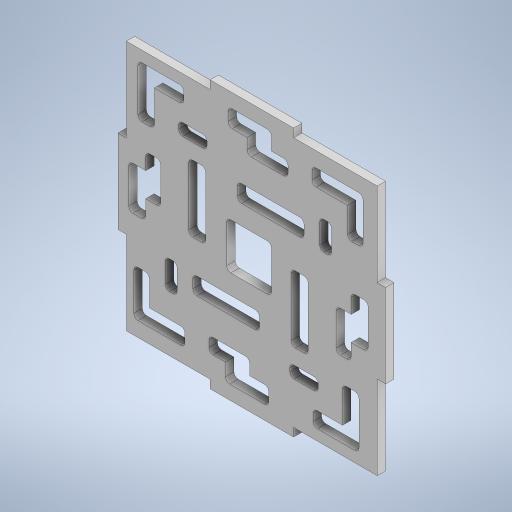
# Autodesk Inventor part: Pièce Ve2
Saved by Autodesk Inventor 2023 (Build 270158000, 158)
## iProperties
Created: 2025-01-14
Part Number: Pièce Ve2
Material: Générique
Document SubType Name: Modeling
Designer: kfadieieva
Density: 1 g/cm^3
Appearance: Par défaut
Author: kfadieieva
Autodesk Inventor part; units mm, degrees
ref_plane "YZ Plane" through (0, 0, 0) normal (1, 0, 0) x (0, 1, 0)
ref_plane "XZ Plane" through (0, 0, 0) normal (0, 1, 0) x (-1, 0, 0)
ref_plane "XY Plane" through (0, 0, 0) normal (0, 0, 1) x (1, 0, 0)
sketch "Esquisse1" plane through (0, 0, 0) normal (0, 0, 1) x (1, 0, 0)
  line L0 (0, 60) -> (-3, 60)
  line L1 (-3, 60) -> (-3, 30)
  line L2 (-3, 30) -> (0, 30)
  line L3 (90, 60) -> (93, 60)
  line L4 (93, 60) -> (93, 30)
  line L5 (93, 30) -> (90, 30)
  line L6 (60, 90) -> (60, 93)
  line L7 (60, 93) -> (30, 93)
  line L8 (30, 93) -> (30, 90)
  line L9 (30, 0) -> (30, -3)
  line L10 (30, -3) -> (60, -3)
  line L11 (60, -3) -> (60, 0)
  line L12 (0, 0) -> (30, 0)
  line L13 (60, 0) -> (90, 0)
  line L14 (90, 90) -> (60, 90)
  line L15 (30, 90) -> (0, 90)
  line L16 (90, 0) -> (90, 30)
  line L17 (90, 60) -> (90, 90)
  line L18 (0, 90) -> (0, 60)
  line L19 (0, 30) -> (0, 0)
  dimension "d0" = 90
  dimension "d1" = 90
  dimension "d6" = 3
  constraints: 40 end point, 13 perpendicular, 8 parallel, 3 equal length, 3 horizontal, 2 point on line, 2 vertical
  measures "d0" distance of L15.end L12.start
  measures "d1" distance of L12.start L13.end
  measures "d6" distance of L0.start L0.end
extrude "Extrusion1" add sketch "Esquisse1" along normal blind 3
sketch "Esquisse2" plane through (0, 0, 3) normal (0, 0, 1) x (1, 0, 0)
  line L0 (5.6535, 86.1061) -> (19.1192, 86.1061)
  line L1 (20.6192, 84.6061) -> (20.6192, 82.0558)
  line L2 (19.1192, 80.5558) -> (10.0738, 80.5558)
  line L3 (4.1535, 80.5558) -> (4.1535, 84.6061)
  line L4 (10.0738, 80.5558) -> (10.0738, 69.2903)
  line L5 (8.5738, 67.7903) -> (5.6535, 67.7903)
  line L6 (4.1535, 69.2903) -> (4.1535, 81.8509)
  line L7 (20.2692, 74.8206) -> (27.4446, 74.8206)
  line L8 (28.9446, 73.3206) -> (28.9446, 72.0654)
  line L9 (27.4446, 70.5654) -> (20.2692, 70.5654)
  line L10 (18.7692, 72.0654) -> (18.7692, 73.3206)
  line L11 (38.0299, 87.9562) -> (50.5706, 87.9562)
  line L12 (52.0706, 86.4562) -> (52.0706, 81.8509)
  line L13 (43.3752, 81.8509) -> (38.0299, 81.8509)
  line L14 (36.5299, 83.3509) -> (36.5299, 86.4562)
  line L15 (52.0706, 81.8509) -> (56.4909, 81.8509)
  line L16 (57.9909, 80.3509) -> (57.9909, 77.9857)
  line L17 (56.4909, 76.4857) -> (44.8752, 76.4857)
  line L18 (43.3752, 77.9857) -> (43.3752, 81.8509)
  arc A0 (5.6535, 86.1061) -> (4.1535, 84.6061) centre (5.6535, 84.6061) ccw
  arc A1 (19.1192, 80.5558) -> (20.6192, 82.0558) centre (19.1192, 82.0558) ccw
  arc A2 (20.6192, 84.6061) -> (19.1192, 86.1061) centre (19.1192, 84.6061) ccw
  arc A3 (20.2692, 74.8206) -> (18.7692, 73.3206) centre (20.2692, 73.3206) ccw
  arc A4 (18.7692, 72.0654) -> (20.2692, 70.5654) centre (20.2692, 72.0654) ccw
  arc A5 (28.9446, 73.3206) -> (27.4446, 74.8206) centre (27.4446, 73.3206) ccw
  arc A6 (27.4446, 70.5654) -> (28.9446, 72.0654) centre (27.4446, 72.0654) ccw
  arc A7 (8.5738, 67.7903) -> (10.0738, 69.2903) centre (8.5738, 69.2903) ccw
  arc A8 (4.1535, 69.2903) -> (5.6535, 67.7903) centre (5.6535, 69.2903) ccw
  arc A9 (43.3752, 77.9857) -> (44.8752, 76.4857) centre (44.8752, 77.9857) ccw
  arc A10 (38.0299, 87.9562) -> (36.5299, 86.4562) centre (38.0299, 86.4562) ccw
  arc A11 (36.5299, 83.3509) -> (38.0299, 81.8509) centre (38.0299, 83.3509) ccw
  arc A12 (56.4909, 76.4857) -> (57.9909, 77.9857) centre (56.4909, 77.9857) ccw
  arc A13 (57.9909, 80.3509) -> (56.4909, 81.8509) centre (56.4909, 80.3509) ccw
  arc A14 (52.0706, 86.4562) -> (50.5706, 87.9562) centre (50.5706, 86.4562) ccw
  line L19 (60, 93) -> (30, 93) projected
  line L20 (93, 30) -> (93, 60) projected
  line L21 (-3, 60) -> (-3, 30) projected
  line L22 (30, -3) -> (60, -3) projected
  line L23 (83.4207, 68.1953) -> (80.8704, 68.1953)
  arc A15 (83.4207, 68.1953) -> (84.9207, 69.6953) centre (83.4207, 69.6953) ccw
  arc A16 (79.3704, 69.6953) -> (80.8704, 68.1953) centre (80.8704, 69.6953) ccw
  line L24 (70.88, 70.0454) -> (72.1352, 70.0454)
  arc A17 (73.6352, 68.5454) -> (72.1352, 70.0454) centre (72.1352, 68.5454) ccw
  arc A18 (70.88, 70.0454) -> (69.38, 68.5454) centre (70.88, 68.5454) ccw
  line L25 (73.6352, 68.5454) -> (73.6352, 61.37)
  line L26 (69.38, 61.37) -> (69.38, 68.5454)
  arc A19 (72.1352, 59.87) -> (73.6352, 61.37) centre (72.1352, 61.37) ccw
  line L27 (72.1352, 59.87) -> (70.88, 59.87)
  arc A20 (69.38, 61.37) -> (70.88, 59.87) centre (70.88, 61.37) ccw
  line L28 (66.6049, 80.2408) -> (66.6049, 83.1611)
  arc A21 (66.6049, 80.2408) -> (68.1049, 78.7408) centre (68.1049, 80.2408) ccw
  arc A22 (68.1049, 84.6611) -> (66.6049, 83.1611) centre (68.1049, 83.1611) ccw
  line L29 (80.6655, 45.4393) -> (80.6655, 50.7846)
  line L30 (80.6655, 36.744) -> (80.6655, 32.3237)
  line L31 (79.1655, 30.8237) -> (76.8002, 30.8237)
  line L32 (75.3002, 32.3237) -> (75.3002, 43.9393)
  line L33 (76.8002, 45.4393) -> (80.6655, 45.4393)
  arc A23 (79.1655, 30.8237) -> (80.6655, 32.3237) centre (79.1655, 32.3237) ccw
  arc A24 (76.8002, 45.4393) -> (75.3002, 43.9393) centre (76.8002, 43.9393) ccw
  arc A25 (75.3002, 32.3237) -> (76.8002, 30.8237) centre (76.8002, 32.3237) ccw
  line L34 (84.9207, 83.1611) -> (84.9207, 69.6953)
  line L35 (79.3704, 69.6953) -> (79.3704, 78.7408)
  line L36 (79.3704, 84.6611) -> (83.4207, 84.6611)
  line L37 (79.3704, 78.7408) -> (68.1049, 78.7408)
  line L38 (68.1049, 84.6611) -> (80.6655, 84.6611)
  arc A26 (84.9207, 83.1611) -> (83.4207, 84.6611) centre (83.4207, 83.1611) ccw
  line L39 (86.7707, 50.7846) -> (86.7707, 38.244)
  line L40 (85.2707, 36.744) -> (80.6655, 36.744)
  line L41 (82.1655, 52.2846) -> (85.2707, 52.2846)
  arc A27 (82.1655, 52.2846) -> (80.6655, 50.7846) centre (82.1655, 50.7846) ccw
  arc A28 (86.7707, 50.7846) -> (85.2707, 52.2846) centre (85.2707, 50.7846) ccw
  arc A29 (85.2707, 36.744) -> (86.7707, 38.244) centre (85.2707, 38.244) ccw
  line L42 (67.0099, 5.3939) -> (67.0099, 7.9442)
  arc A30 (67.0099, 5.3939) -> (68.5099, 3.8939) centre (68.5099, 5.3939) ccw
  arc A31 (68.5099, 9.4442) -> (67.0099, 7.9442) centre (68.5099, 7.9442) ccw
  line L43 (68.86, 17.9346) -> (68.86, 16.6794)
  arc A32 (67.36, 15.1794) -> (68.86, 16.6794) centre (67.36, 16.6794) ccw
  arc A33 (68.86, 17.9346) -> (67.36, 19.4346) centre (67.36, 17.9346) ccw
  line L44 (67.36, 15.1794) -> (60.1846, 15.1794)
  line L45 (60.1846, 19.4346) -> (67.36, 19.4346)
  arc A34 (58.6846, 16.6794) -> (60.1846, 15.1794) centre (60.1846, 16.6794) ccw
  line L46 (58.6846, 16.6794) -> (58.6846, 17.9346)
  arc A35 (60.1846, 19.4346) -> (58.6846, 17.9346) centre (60.1846, 17.9346) ccw
  line L47 (79.0554, 22.2097) -> (81.9756, 22.2097)
  arc A36 (79.0554, 22.2097) -> (77.5554, 20.7097) centre (79.0554, 20.7097) ccw
  arc A37 (83.4756, 20.7097) -> (81.9756, 22.2097) centre (81.9756, 20.7097) ccw
  line L48 (44.2539, 8.1491) -> (49.5992, 8.1491)
  line L49 (35.5585, 8.1491) -> (31.1383, 8.1491)
  line L50 (29.6383, 9.6491) -> (29.6383, 12.0143)
  line L51 (31.1383, 13.5143) -> (42.7539, 13.5143)
  line L52 (44.2539, 12.0143) -> (44.2539, 8.1491)
  arc A38 (29.6383, 9.6491) -> (31.1383, 8.1491) centre (31.1383, 9.6491) ccw
  arc A39 (44.2539, 12.0143) -> (42.7539, 13.5143) centre (42.7539, 12.0143) ccw
  arc A40 (31.1383, 13.5143) -> (29.6383, 12.0143) centre (31.1383, 12.0143) ccw
  line L53 (81.9756, 3.8939) -> (68.5099, 3.8939)
  line L54 (68.5099, 9.4442) -> (77.5554, 9.4442)
  line L55 (83.4756, 9.4442) -> (83.4756, 5.3939)
  line L56 (77.5554, 9.4442) -> (77.5554, 20.7097)
  line L57 (83.4756, 20.7097) -> (83.4756, 8.1491)
  arc A41 (81.9756, 3.8939) -> (83.4756, 5.3939) centre (81.9756, 5.3939) ccw
  line L58 (49.5992, 2.0438) -> (37.0585, 2.0438)
  line L59 (35.5585, 3.5438) -> (35.5585, 8.1491)
  line L60 (51.0992, 6.6491) -> (51.0992, 3.5438)
  arc A42 (51.0992, 6.6491) -> (49.5992, 8.1491) centre (49.5992, 6.6491) ccw
  arc A43 (49.5992, 2.0438) -> (51.0992, 3.5438) centre (49.5992, 3.5438) ccw
  arc A44 (35.5585, 3.5438) -> (37.0585, 2.0438) centre (37.0585, 3.5438) ccw
  line L61 (4.2085, 21.8047) -> (6.7587, 21.8047)
  arc A45 (4.2085, 21.8047) -> (2.7085, 20.3047) centre (4.2085, 20.3047) ccw
  arc A46 (8.2587, 20.3047) -> (6.7587, 21.8047) centre (6.7587, 20.3047) ccw
  line L62 (16.7492, 19.9546) -> (15.494, 19.9546)
  arc A47 (13.994, 21.4546) -> (15.494, 19.9546) centre (15.494, 21.4546) ccw
  arc A48 (16.7492, 19.9546) -> (18.2492, 21.4546) centre (16.7492, 21.4546) ccw
  line L63 (13.994, 21.4546) -> (13.994, 28.63)
  line L64 (18.2492, 28.63) -> (18.2492, 21.4546)
  arc A49 (15.494, 30.13) -> (13.994, 28.63) centre (15.494, 28.63) ccw
  line L65 (15.494, 30.13) -> (16.7492, 30.13)
  arc A50 (18.2492, 28.63) -> (16.7492, 30.13) centre (16.7492, 28.63) ccw
  line L66 (21.0243, 9.7592) -> (21.0243, 6.8389)
  arc A51 (21.0243, 9.7592) -> (19.5243, 11.2592) centre (19.5243, 9.7592) ccw
  arc A52 (19.5243, 5.3389) -> (21.0243, 6.8389) centre (19.5243, 6.8389) ccw
  line L67 (6.9637, 44.5607) -> (6.9637, 39.2154)
  line L68 (6.9637, 53.256) -> (6.9637, 57.6763)
  line L69 (8.4637, 59.1763) -> (10.8289, 59.1763)
  line L70 (12.3289, 57.6763) -> (12.3289, 46.0607)
  line L71 (10.8289, 44.5607) -> (6.9637, 44.5607)
  arc A53 (8.4637, 59.1763) -> (6.9637, 57.6763) centre (8.4637, 57.6763) ccw
  arc A54 (10.8289, 44.5607) -> (12.3289, 46.0607) centre (10.8289, 46.0607) ccw
  arc A55 (12.3289, 57.6763) -> (10.8289, 59.1763) centre (10.8289, 57.6763) ccw
  line L72 (2.7085, 6.8389) -> (2.7085, 20.3047)
  line L73 (8.2587, 20.3047) -> (8.2587, 11.2592)
  line L74 (8.2587, 5.3389) -> (4.2085, 5.3389)
  line L75 (8.2587, 11.2592) -> (19.5243, 11.2592)
  line L76 (19.5243, 5.3389) -> (6.9637, 5.3389)
  arc A56 (2.7085, 6.8389) -> (4.2085, 5.3389) centre (4.2085, 6.8389) ccw
  line L77 (0.8584, 39.2154) -> (0.8584, 51.756)
  line L78 (2.3584, 53.256) -> (6.9637, 53.256)
  line L79 (5.4637, 37.7154) -> (2.3584, 37.7154)
  arc A57 (5.4637, 37.7154) -> (6.9637, 39.2154) centre (5.4637, 39.2154) ccw
  arc A58 (0.8584, 39.2154) -> (2.3584, 37.7154) centre (2.3584, 39.2154) ccw
  arc A59 (2.3584, 53.256) -> (0.8584, 51.756) centre (2.3584, 51.756) ccw
  line L80 (37.4979, 53.256) -> (50.5706, 53.256)
  line L81 (52.0706, 51.756) -> (52.0706, 38.244)
  line L82 (50.5706, 36.744) -> (37.4979, 36.744)
  line L83 (35.9979, 38.244) -> (35.9979, 51.756)
  line L84 (23.8699, 41.0533) -> (27.0053, 41.0533)
  line L85 (28.5053, 42.5533) -> (28.5053, 63.4577)
  line L86 (27.0053, 64.9577) -> (23.8699, 64.9577)
  line L87 (22.3699, 63.4577) -> (22.3699, 42.5533)
  arc A60 (23.8699, 64.9577) -> (22.3699, 63.4577) centre (23.8699, 63.4577) ccw
  arc A61 (28.5053, 63.4577) -> (27.0053, 64.9577) centre (27.0053, 63.4577) ccw
  arc A62 (27.0053, 41.0533) -> (28.5053, 42.5533) centre (27.0053, 42.5533) ccw
  arc A63 (22.3699, 42.5533) -> (23.8699, 41.0533) centre (23.8699, 42.5533) ccw
  arc A64 (37.4979, 53.256) -> (35.9979, 51.756) centre (37.4979, 51.756) ccw
  arc A65 (52.0706, 51.756) -> (50.5706, 53.256) centre (50.5706, 51.756) ccw
  arc A66 (50.5706, 36.744) -> (52.0706, 38.244) centre (50.5706, 38.244) ccw
  arc A67 (35.9979, 38.244) -> (37.4979, 36.744) centre (37.4979, 38.244) ccw
  arc A68 (63.7723, 64.9446) -> (62.2723, 66.4446) centre (62.2723, 64.9446) ccw
  line L88 (63.7723, 61.8093) -> (63.7723, 64.9446)
  arc A69 (62.2723, 60.3093) -> (63.7723, 61.8093) centre (62.2723, 61.8093) ccw
  line L89 (62.2723, 66.4446) -> (41.3679, 66.4446)
  line L90 (41.3679, 60.3093) -> (62.2723, 60.3093)
  arc A70 (41.3679, 66.4446) -> (39.8679, 64.9446) centre (41.3679, 64.9446) ccw
  line L91 (39.8679, 64.9446) -> (39.8679, 61.8093)
  arc A71 (39.8679, 61.8093) -> (41.3679, 60.3093) centre (41.3679, 61.8093) ccw
  arc A72 (63.7592, 25.0423) -> (65.2592, 26.5423) centre (63.7592, 26.5423) ccw
  line L92 (60.6239, 25.0423) -> (63.7592, 25.0423)
  arc A73 (59.1239, 26.5423) -> (60.6239, 25.0423) centre (60.6239, 26.5423) ccw
  line L93 (65.2592, 26.5423) -> (65.2592, 47.4467)
  line L94 (59.1239, 47.4467) -> (59.1239, 26.5423)
  arc A74 (65.2592, 47.4467) -> (63.7592, 48.9467) centre (63.7592, 47.4467) ccw
  line L95 (63.7592, 48.9467) -> (60.6239, 48.9467)
  arc A75 (60.6239, 48.9467) -> (59.1239, 47.4467) centre (60.6239, 47.4467) ccw
  arc A76 (23.8569, 25.0554) -> (25.3569, 23.5554) centre (25.3569, 25.0554) ccw
  line L96 (23.8569, 28.1907) -> (23.8569, 25.0554)
  arc A77 (25.3569, 29.6907) -> (23.8569, 28.1907) centre (25.3569, 28.1907) ccw
  line L97 (25.3569, 23.5554) -> (46.2613, 23.5554)
  line L98 (46.2613, 29.6907) -> (25.3569, 29.6907)
  arc A78 (46.2613, 23.5554) -> (47.7613, 25.0554) centre (46.2613, 25.0554) ccw
  line L99 (47.7613, 25.0554) -> (47.7613, 28.1907)
  arc A79 (47.7613, 28.1907) -> (46.2613, 29.6907) centre (46.2613, 28.1907) ccw
  point P0 (0, 0)
  point P1 (45, 93)
  point P2 (93, 45)
  point P3 (-3, 45)
  point P4 (45, -3)
  point P5 (43.8146, 45)
  dimension "d9" = 1.5
  dimension "d10" = 1.5
  dimension "d13" = 360
  dimension "d15" = 1.5
  dimension "d18" = 360
  constraints: 192 end point, 160 point on circle, 80 centre point, 46 tangent, 20 equal radius, 13 parallel, 6 horizontal, 6 perpendicular, 4 midpoint, 4 point on line, 418 other
  measures "d9" radius of A0
  measures "d10" radius of A12
  measures "d15" radius of A60
extrude "Extrusion2" cut sketch "Esquisse2" against normal through all
